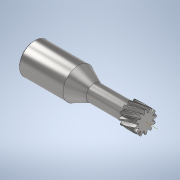
# Autodesk Inventor part: Валл быстроходный
Saved by Autodesk Inventor 2021.2 (Build 252289000, 289)
## iProperties
Created: 2023-03-09
Part Number: Валл быстроходный
Material: Сталь, углеродистая
Document SubType Name: Modeling
Designer: gdevc
Density: 7.85 g/cm^3
Appearance: С умеренной полировкой
Mass: 704.204 g
Surface Area: 248.422 cm^2
Volume: 89.7075 cm^3
Author: gdevc
Autodesk Inventor part; units mm, degrees
ref_plane "YZ Plane" through (0, 0, 0) normal (1, 0, 0) x (0, 1, 0)
ref_plane "XZ Plane" through (0, 0, 0) normal (0, 1, 0) x (-1, 0, 0)
ref_plane "XY Plane" through (0, 0, 0) normal (0, 0, 1) x (1, 0, 0)
sketch "Эскиз1" plane through (0, 0, 0) normal (0, 0, 1) x (1, 0, 0)
  line L0 (0, 14) -> (0, 21)
  line L1 (0, 21) -> (60, 21)
  line L2 (60, 21) -> (81.4451, 11)
  line L3 (81.4451, 11) -> (129.4451, 11)
  line L4 (151.4451, 11) -> (151.4451, 0)
  line L5 (151.4451, 0) -> (0, 0) construction
  line L6 (0, 14) -> (60, 14)
  line L7 (60, 14) -> (60, 0)
  line L8 (60, 14) -> (68.0829, 0)
  line L9 (68.0829, 0) -> (60, 0)
  line L10 (68.0829, 0) -> (151.4451, 0)
  line L11 (151.4451, 11) -> (151.4451, 15.6)
  line L12 (151.4451, 15.6) -> (129.4451, 15.6)
  line L13 (129.4451, 15.6) -> (129.4451, 11)
  dimension "d1" = 42
  dimension "d2" = 30
  dimension "d3" = 28
  dimension "d4" = 60
  dimension "d5" = 25
  dimension "d6" = 70
  dimension "d14" = 22
  dimension "d15" = 31.2
  dimension "d16" = 22
  constraints: 28 end point, 4 perpendicular, 3 horizontal, 3 vertical, 2 point on line, 2 vertical alignment, 1 collinear
  measures "d1" diameter of L1 L5
  measures "d2" angle of L7 L8
  measures "d3" diameter of L6 L5
  measures "d4" distance of L0.start L6.end
  measures "d5" angle of L3 L2
  measures "d6" distance from line of L2.end L4
  measures "d14" diameter of L3 L5
  measures "d15" diameter of L12 L5
  measures "d16" distance between parallel lines of L11 L13
revolve "Вращение1" add sketch "Эскиз1" angle 360 about axis through (151.4451, 0, 0) along (-1, 0, 0) contours L0 L1 L2 L3 L13 L12 L11 L4 L10 L8 L6
sketch "Эскиз2" plane through (0, 0, 0) normal (-1, 0, 0) x (0, 0, 1)
  circle A0 centre (0, 0) radius 14 projected
  line L0 (-4, 17.3) -> (4, 17.3)
  line L1 (4, 17.3) -> (4, 10)
  line L2 (4, 10) -> (-4, 10)
  line L3 (-4, 10) -> (-4, 17.3)
  point P0 (0, 17.3)
  point P1 (-4, 13.4164)
  point P2 (4, 13.4164)
  dimension "d8" = 8
  dimension "d9" = 7.3
  dimension "d11" = 4
  constraints: 8 end point, 2 parallel, 1 horizontal, 1 midpoint, 1 perpendicular, 1 vertical alignment
  measures "d8" distance of L0.start L0.end
  measures "d9" distance between parallel lines of L2 L0
  measures "d11" distance edge to line of A0 L2
extrude "Выдавливание1" cut sketch "Эскиз2" against normal blind 60 contours A0 L3 L0 L1
spur gear teeth "Цилиндрическое зубчатое зацепление1" teeth 12 pitch diameter 25.2 tip diameter 29.2 root diameter 20.2 face width 22 helix angle 17.753 hand left trims to tip circle yes start plane through (151.4451, 0, 0) normal (1, 0, 0) x (0, 1, 0)
chamfer "Фаска1" distance 1 angle 45 5 edges at (0, -21, 0) (0, 15.3582, -4) (0, 17.3, 0) (0, 15.3582, 4) (0, -14, 0)
